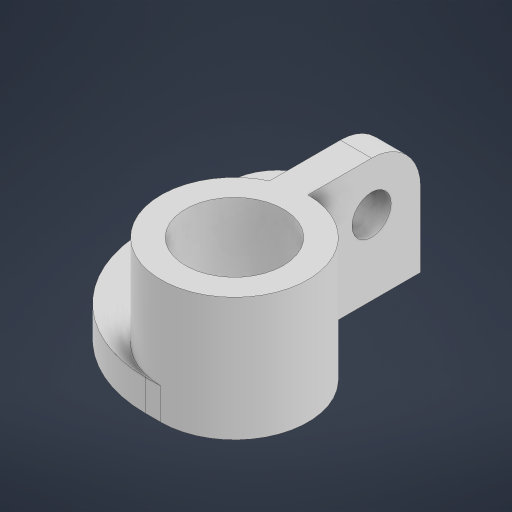
# Autodesk Inventor part: Część1
Saved by Autodesk Inventor 2023 (Build 270158000, 158)
## iProperties
Created: 2023-05-07
Part Number: Część1
Material: Ogólny
Document SubType Name: Modeling
Designer: Adam
Density: 1 g/cm^3
Appearance: Domyślna
Author: Adam
Autodesk Inventor part; units mm, degrees
ref_plane "YZ Plane" through (0, 0, 0) normal (1, 0, 0) x (0, 1, 0)
ref_plane "XZ Plane" through (0, 0, 0) normal (0, 1, 0) x (-1, 0, 0)
ref_plane "XY Plane" through (0, 0, 0) normal (0, 0, 1) x (1, 0, 0)
sketch "Szkic1" plane through (0, 0, 0) normal (0, 1, 0) x (-1, 0, 0)
  line L0 (-65, 0) -> (-73, 0)
  line L1 (-73, 0) -> (-73, -132.5)
  line L2 (-73, -132.5) -> (-25, -132.5)
  line L3 (0, -107.5) -> (0, -65)
  arc A0 (-25, -132.5) -> (0, -107.5) centre (-25, -107.5) ccw
  arc A1 (0, -65) -> (-65, 0) centre (-65, -65) ccw
  circle A2 centre (-73, -37.5) radius 37.5
  point P0 (0, 0)
  point P1 (0, -132.5)
  point P2 (-73, -75)
  dimension "d4" = 75
  dimension "d0" = 73
  dimension "d1" = 132.5
  dimension "d2" = 25
  dimension "d3" = 65
  constraints: 8 end point, 5 point on line, 4 point on circle, 4 tangent, 2 centre point, 2 parallel, 1 horizontal, 1 perpendicular, 3 other
  measures "d0" distance of point (0, -132.5) L1.end
  measures "d1" distance of L1.end L0.end
  measures "d2" radius of A0
  measures "d3" radius of A1
extrude "Wyciągnięcie proste1" add sketch "Szkic1" along normal blind 16 contours A1 L3 A0 L2 L1 A2 L0
sketch "Szkic2" plane through (0, 0, 0) normal (0, -1, 0) x (1, 0, 0)
  arc A0 (73, 0) -> (73, -75) centre (73, -37.5) ccw projected
  circle A1 centre (73, -37.5) radius 37.5
  point P0 (0, 0)
  point P1 (73, -75)
  constraints: 1 centre point, 1 coincident
extrude "Wyciągnięcie proste2" add sketch "Szkic2" against normal blind 63
sketch "Szkic3" plane through (0, 16, 0) normal (0, 1, 0) x (1, 0, 0)
  arc A0 (25, 132.5) -> (0, 107.5) centre (25, 107.5) ccw projected
  line L0 (73, 132.5) -> (25, 132.5) projected
  line L1 (73, 75) -> (73, 132.5) projected
  line L2 (73, 132.5) -> (73, 75)
  line L3 (73, 132.5) -> (57, 132.5)
  line L4 (57, 132.5) -> (57, 71.4153)
  arc A1 (73, 75) -> (73, 0) centre (73, 37.5) ccw projected
  arc A2 (73, 75) -> (57, 71.4153) centre (73, 37.5) ccw
  point P0 (0, 0)
  dimension "d9" = 16
  constraints: 6 end point, 3 point on circle, 1 centre point, 1 coincident, 1 concentric, 1 perpendicular, 1 point on line
  measures "d9" distance of L0.start L3.end
extrude "Wyciągnięcie proste3" add sketch "Szkic3" along normal blind 47
fillet "Zaokrąglenie1" radius 25 1 edges at (65, 63, -132.5)
sketch "Szkic4" plane through (0, 63, 0) normal (0, 1, 0) x (1, 0, 0)
  arc A0 (57, 71.4153) -> (73, 0) centre (73, 37.5) ccw projected
  point P0 (0, 0)
  constraints: 1 coincident
hole "Otwór1" at (73, 63, -37.5) direction (0, -1, 0) diameter 50 end through all
sketch "Szkic5" plane through (57, 16, -132.5) normal (-1, 0, 0) x (0, 0, 1)
  arc A0 (25, 47) -> (0, 22) centre (25, 22) ccw projected
  point P0 (132.5, -16)
  constraints: 1 coincident
hole "Otwór2" at (57, 38, -107.5) direction (1, 0, 0) diameter 20 end through all
sketch "Szkic6" plane through (0, 16, 0) normal (0, 1, 0) x (1, 0, 0)
  arc A0 (25, 132.5) -> (0, 107.5) centre (25, 107.5) ccw projected
  point P0 (0, 0)
  constraints: 1 coincident
hole "Otwór3" at (25, 16, -107.5) direction (0, -1, 0) diameter 22 end through all
